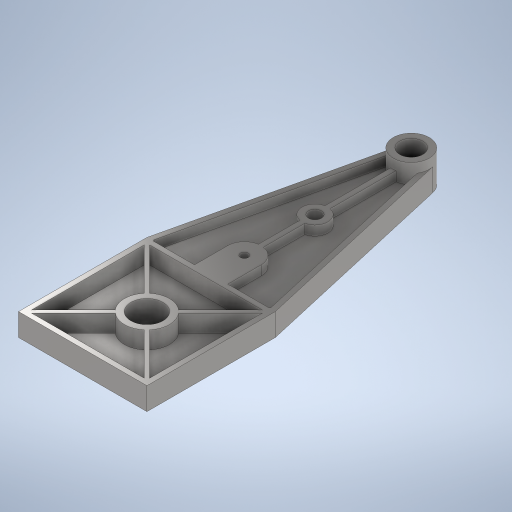
# Autodesk Inventor part: boat
Saved by Autodesk Inventor 2024 (Build 280153000, 153)
## iProperties
Created: 2024-02-02
Part Number: boat
Material: Stahl, galvanisiert
Document SubType Name: Modeling
Designer: ffogue
Density: 7.85 g/cm^3
Appearance: Galvanisiert
Author: ffogue
Autodesk Inventor part; units mm, degrees
ref_plane "XY Plane" through (0, 0, 0) normal (0, 0, 1) x (1, 0, 0)
sketch "Skizze1" plane through (0, 0, 0) normal (0, 0, 1) x (1, 0, 0)
  line L0 (-100, 0) -> (100, 0)
  line L1 (100, 0) -> (100, 200)
  circle A0 centre (0, 511.7594) radius 28
  line L2 (-27.2957, 518) -> (-100, 200)
  line L3 (-100, 200) -> (-100, 0)
  line L4 (0, 511.7594) -> (0, 0) construction
  circle A1 centre (0, 511.7594) radius 18
  line L5 (100, 200) -> (27.2957, 518)
  point P0 (27.2957, 518)
  dimension "d0" = 56
  dimension "d1" = 36
  dimension "d2" = 518
  dimension "d3" = 200
  dimension "d4" = 200
  dimension "d8" = 318
  constraints: 12 end point, 3 perpendicular, 3 point on circle, 2 centre point, 2 coincident, 2 midpoint, 2 tangent, 1 horizontal, 1 parallel, 1 symmetric about line, 1 other
  measures "d0" diameter of A0
  measures "d1" diameter of A1
  measures "d2" distance from line of L0 A0.end
  measures "d3" distance of L0.start L2.end
  measures "d4" distance between parallel lines of L1 L3
  measures "d8" vertical distance of L1.end L5.end
extrude "Extrusion1" add sketch "Skizze1" along normal blind 50 contours A0
extrude "Extrusion2" add sketch "Skizze1" along normal blind 35 contours L3 L2 A0 L5 L1 L0
sketch "Skizze6" plane through (0, 0, 35) normal (0, 0, 1) x (1, 0, 0)
  line L0 (-100, 200) -> (-100, 0) projected
  line L1 (100, 0) -> (100, 200) projected
  line L2 (-100, 0) -> (100, 0) projected
  line L3 (0, 0) -> (0, 223.6261) construction
  line L4 (100, 100) -> (-100, 100) construction
  line L5 (0, 100) -> (-100, 200) construction
  circle A0 centre (0, 100) radius 35
  line L6 (-92, 8) -> (92, 8)
  line L7 (92, 8) -> (92, 192)
  line L8 (92, 192) -> (-92, 192)
  line L9 (-92, 192) -> (-92, 8)
  line L10 (-26.779, 122.5363) -> (-92, 187.7574)
  line L11 (-22.5363, 126.779) -> (-87.7574, 192)
  line L12 (0, 100) -> (-92, 8) construction
  line L13 (-22.5363, 73.221) -> (-87.7574, 8)
  line L14 (-26.779, 77.4637) -> (-92, 12.2426)
  line L15 (0, 100) -> (92, 8) construction
  line L16 (26.779, 77.4637) -> (92, 12.2426)
  line L17 (22.5363, 73.221) -> (87.7574, 8)
  point P0 (0, 8)
  point P1 (0, 0)
  dimension "d36" = 100
  dimension "d37" = 70
  dimension "d38" = 8
  dimension "d39" = 8
  dimension "d40" = 8
  dimension "d41" = 6
  dimension "d42" = 45
  dimension "d43" = 6
  dimension "d47" = 6
  constraints: 30 end point, 10 parallel, 7 point on line, 6 point on circle, 5 midpoint, 2 perpendicular, 1 centre point, 1 coincident, 1 horizontal, 1 vertical, 1 vertical alignment, 1 other
  measures "d36" distance between parallel lines of L2 L4
  measures "d37" diameter of A0
  measures "d38" distance from line of L1.end L8
  measures "d39" distance between parallel lines of L1 L7
  measures "d40" distance between parallel lines of L2 L6
  measures "d41" distance between parallel lines of L11 L10
  measures "d42" angle of L3 L12
  measures "d43" distance between parallel lines of L13 L14
  measures "d47" distance between parallel lines of L17 L16
ref_plane "Arbeitsebene1" through (0, 0, 0) normal (1, 0, 0) x (0, 1, 0)
extrude "Extrusion8" cut sketch "Skizze6" against normal blind 27 contours A0 L14 L9 L10
extrude "Extrusion9" cut sketch "Skizze6" against normal blind 27 contours L17 L6 L13 A0
mirror "Spiegeln2" about plane through (0, 0, 0) normal (1, 0, 0) of "Extrusion8"
ref_plane "Arbeitsebene2" through (0, 100, 0) normal (0, 1, 0) x (-1, 0, 0)
mirror "Spiegeln3" about plane through (0, 100, 0) normal (0, 1, 0) of "Extrusion9"
sketch "Skizze7" plane through (0, 0, 35) normal (0, 0, 1) x (1, 0, 0)
  circle A0 centre (0, 100) radius 25
  line L0 (-100, 0) -> (100, 0) projected
  point P0 (0, 0)
  point P1 (0, 0)
  point P2 (0, 0)
  dimension "d53" = 50
  dimension "d54" = 100
  constraints: 2 midpoint, 1 centre point, 1 vertical alignment
  measures "d53" diameter of A0
  measures "d54" distance of point (0, 0) A0.centre
extrude "Extrusion10" cut sketch "Skizze7" against normal up to surface (35 mm away)
sketch "Skizze8" plane through (0, 0, 35) normal (0, 0, 1) x (1, 0, 0)
  line L0 (-87.7574, 192) -> (87.7574, 192) projected
  circle A0 centre (0, 511.7594) radius 28 projected
  line L1 (91.7936, 200) -> (23.8644, 497.114)
  line L2 (-91.7936, 200) -> (-23.8644, 497.114)
  line L3 (-27.2957, 518) -> (-100, 200) projected
  line L4 (100, 200) -> (27.2957, 518) projected
  arc A1 (26, 251.7594) -> (-26, 251.7594) centre (0, 251.7594) ccw
  line L5 (-26, 251.7594) -> (-26, 200)
  line L6 (26, 251.7594) -> (26, 200)
  line L7 (0, 511.7594) -> (0, 277.7594) construction
  line L8 (-91.7936, 200) -> (-26, 200)
  line L9 (26, 200) -> (91.7936, 200)
  line L10 (-100, 0) -> (100, 0) projected
  circle A2 centre (0, 361.7594) radius 20
  line L11 (-4, 277.4499) -> (-4, 342.1635)
  line L12 (4, 277.4499) -> (4, 342.1635)
  line L13 (-4, 381.3553) -> (-4, 484.0466)
  line L14 (4, 381.3553) -> (4, 484.0466)
  point P0 (0, 0)
  point P1 (0, 0)
  dimension "d57" = 8
  dimension "d60" = 8
  dimension "d64" = 260
  dimension "d65" = 26
  dimension "d66" = 40
  dimension "d67" = 110
  dimension "d68" = 8
  constraints: 22 end point, 13 point on circle, 5 point on line, 4 parallel, 4 perpendicular, 2 centre point, 2 equal length, 2 horizontal alignment, 2 vertical, 1 midpoint, 1 vertical alignment, 2 other
  measures "d57" distance between parallel lines of L2 L3
  measures "d60" distance between parallel lines of L0 L9
  measures "d64" distance of A1.centre L7.start
  measures "d65" radius of A1
  measures "d66" diameter of A2
  measures "d67" distance of A1.centre A2.centre
  measures "d68" distance between parallel lines of L12 L11
extrude "Extrusion11" cut sketch "Skizze8" against normal blind 15 contours L1 L9 L6 A1 L12 A2 L14 A0 | A0 L13 A2 L11 A1 L5 L8 L2
sketch "Skizze9" plane through (0, 0, 35) normal (0, 0, 1) x (1, 0, 0)
  arc A0 (26, 251.7594) -> (4, 277.4499) centre (0, 251.7594) ccw projected
  point P0 (0, 0)
  constraints: 1 coincident
hole "Bohrung1" at (0, 251.7594, 35) direction (0, 0, -1) diameter 12 depth 35
sketch "Skizze10" plane through (0, 0, 35) normal (0, 0, 1) x (1, 0, 0)
  arc A0 (-4, 381.3553) -> (-4, 342.1635) centre (0, 361.7594) ccw projected
  point P0 (0, 0)
  constraints: 1 coincident
hole "Bohrung2" at (0, 361.7594, 35) direction (0, 0, -1) diameter 20 depth 35
fillet "Rundung1" radius 2 2 edges at (-91.7936, 200, 27.5) (91.7936, 200, 27.5)
equation "\"d43\" = d41"
equation "\"d47\" = d41"
